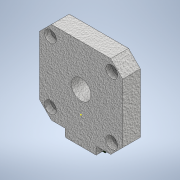
# Autodesk Inventor part: Part1
Saved by Autodesk Inventor 2021 (Build 250183000, 183)
## iProperties
Created: 2020-06-30
Part Number: Part1
Material: Genérico
Document SubType Name: Modeling
Designer: IVAN
Density: 1 g/cm^3
Appearance: Por defecto
Author: IVAN
Autodesk Inventor part; units mm, degrees
ref_plane "YZ Plane" through (0, 0, 0) normal (1, 0, 0) x (0, 1, 0)
ref_plane "XZ Plane" through (0, 0, 0) normal (0, 1, 0) x (-1, 0, 0)
ref_plane "XY Plane" through (0, 0, 0) normal (0, 0, 1) x (1, 0, 0)
sketch "Sketch1" plane through (0, 0, 0) normal (0, 1, 0) x (-1, 0, 0)
  line L0 (-21, -21) -> (21, -21)
  line L1 (21, -21) -> (21, 21)
  line L2 (21, 21) -> (-21, 21)
  line L3 (-21, 21) -> (-21, -21)
  line L4 (-21, -21) -> (21, 21) construction
  line L5 (21, -21) -> (-21, 21) construction
  point P0 (0, 0)
  dimension "d0" = 42
  dimension "d1" = 42
  constraints: 12 end point, 2 midpoint, 2 parallel, 1 horizontal, 1 perpendicular
  measures "d0" distance of L2.end L1.end
  measures "d1" distance of L1.end L0.end
extrude "Extrusion1" add sketch "Sketch1" along normal blind 9
chamfer "Chamfer1" distance 6 angle 45 4 edges at (21, 4.5, -21) (-21, 4.5, -21) (-21, 4.5, 21) (21, 4.5, 21)
sketch "Sketch2" plane through (0, 9, 0) normal (0, 1, 0) x (1, 0, 0)
  point P0 (0, 0)
sketch "Sketch3" plane through (0, 0, 0) normal (0, -1, 0) x (1, 0, 0)
  circle A0 centre (0, 0) radius 5
  dimension "d7" = 10
  constraints: 1 centre point, 1 coincident
  measures "d7" diameter of A0
extrude "Extrusion2" cut sketch "Sketch3" against normal up to surface (9 mm away)
sketch "Sketch4" plane through (0, 9, 0) normal (0, 1, 0) x (1, 0, 0)
  circle A0 centre (-15.5, -15.5) radius 1.5
  line L0 (-15, -21) -> (15, -21) projected
  line L1 (-21, 15) -> (-21, -15) projected
  point P0 (0, 0)
  dimension "d10" = 3
  dimension "d11" = 5.5
  dimension "d12" = 5.5
  constraints: 1 centre point
  measures "d10" diameter of A0
  measures "d11" distance from line of L0 A0.centre
  measures "d12" distance from line of L1 A0.centre
extrude "Extrusion3" cut sketch "Sketch4" against normal up to surface (9 mm away)
mirror "Mirror1" about plane through (0, 0, 0) normal (1, 0, 0) of "Extrusion3"
mirror "Mirror2" about plane through (0, 0, 0) normal (0, 0, 1) of "Extrusion3", "Mirror1"
sketch "Sketch6" plane through (0, 0, 0) normal (0, -1, 0) x (1, 0, 0)
  circle A0 centre (15.5, -15.5) radius 1.5 projected
  circle A1 centre (-15.5, -15.5) radius 1.5 projected
  circle A2 centre (15.5, 15.5) radius 1.5 projected
  circle A3 centre (-15.5, 15.5) radius 1.5 projected
  circle A4 centre (0, 0) radius 5 projected
  line L0 (15, 21) -> (21, 15) projected
  line L1 (-15, 21) -> (15, 21) projected
  line L2 (-21, 15) -> (-15, 21) projected
  line L3 (-21, -15) -> (-21, 15) projected
  line L4 (-15, -21) -> (-21, -15) projected
  line L5 (15, -21) -> (-15, -21) projected
  line L6 (21, -15) -> (15, -21) projected
  line L7 (21, 15) -> (21, -15) projected
  line L8 (8, -21) -> (-8, -21)
  line L9 (-8, -21) -> (-8, -25)
  line L10 (-8, -25) -> (8, -25)
  line L11 (8, -25) -> (8, -21)
  dimension "d20" = 16
  dimension "d21" = 8
  dimension "d24" = 4
  constraints: 8 end point, 2 parallel, 1 horizontal, 1 perpendicular, 1 point on line
  measures "d20" distance of L9.end L10.end
  measures "d21" distance from line of point (0, 0) L9
  measures "d24" distance of L8.end L9.end
extrude "Extrusion5" add sketch "Sketch6" against normal blind 4 contours L11 L10 L9 L5
fillet "Fillet1" radius 0.5 2 edges at (8, 2, -25) (-8, 2, -25)
sketch "Sketch7" plane through (15, 9, -21) normal (0, 0, -1) x (-1, 0, 0)
  line L0 (23, -5) -> (23, -9) projected
  line L1 (23, -9) -> (30, -9) projected
  line L2 (30, 0) -> (30, -9) projected
  line L3 (0, 0) -> (30, 0) projected
  line L4 (0, -9) -> (0, 0) projected
  line L5 (0, -9) -> (7, -9) projected
  line L6 (7, -9) -> (7, -5) projected
  line L7 (7, -5) -> (23, -5) projected
  line L8 (7, -5) -> (23, -5)
  line L9 (23, -5) -> (23, 0)
  line L10 (23, 0) -> (7, 0)
  line L11 (7, 0) -> (7, -5)
  point P0 (15, -9)
  constraints: 8 end point, 2 parallel, 1 collinear, 1 horizontal, 1 perpendicular
extrude "Extrusion6" cut sketch "Sketch7" against normal blind 10 contours L7 L11 L3 L9
sketch "Sketch8" plane through (15, 9, -11) normal (0, 0, -1) x (-1, 0, 0)
  line L0 (23, -5) -> (7, -5) projected
  line L1 (23, 0) -> (23, -5) projected
  line L2 (7, 0) -> (23, 0) projected
  line L3 (7, -5) -> (7, 0) projected
  line L4 (23, 0) -> (23, -5) projected
  line L5 (7, -4.3) -> (23, -4.3)
  line L6 (23, -4.3) -> (23, -4.8)
  line L7 (23, -4.8) -> (7, -4.8)
  line L8 (7, -4.8) -> (7, -4.3)
  point P0 (15, -9)
  dimension "d28" = 0.5
  dimension "d29" = 0.2
  constraints: 8 end point, 2 parallel, 2 point on line, 1 horizontal, 1 perpendicular
  measures "d28" distance between parallel lines of L7 L5
  measures "d29" distance between parallel lines of L0 L7
extrude "Extrusion7" add sketch "Sketch8" along normal blind 15 contours L7 L3 L5 L1
sketch "Sketch9" plane through (15, 9, -11) normal (0, 0, -1) x (-1, 0, 0)
  point P0 (15, -9)
sketch "Sketch10" plane through (0, 0, 0) normal (0, -1, 0) x (1, 0, 0)
  circle A0 centre (15.5, 15.5) radius 1.5 projected
  circle A1 centre (15.5, 15.5) radius 3
  point P0 (0, 0)
  dimension "d32" = 6
  constraints: 1 centre point, 1 coincident
  measures "d32" diameter of A1
extrude "Extrusion8" cut sketch "Sketch10" against normal blind 3
mirror "Mirror3" about plane through (0, 0, 0) normal (1, 0, 0) of "Extrusion8"
mirror "Mirror4" about plane through (0, 0, 0) normal (0, 0, 1) of "Extrusion8", "Mirror3"
equation "\"d12\" = d11"
equation "\"d21\" = 0.5 * d20"
body "Solid1"
